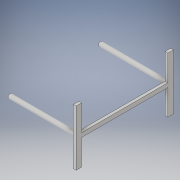
# Autodesk Inventor part: Spielstraßenschild_Teil_Unten
Saved by Autodesk Inventor 2019.5 (Build 235369000, 369)
## iProperties
Created: 2021-10-06
Part Number: Spielstraßenschild_Teil_Unten
Material: Generisch
Document SubType Name: Modeling
Designer: mritt
Density: 1 g/cm^3
Appearance: Vorgabe
Author: mritt
Autodesk Inventor part; units mm, degrees
ref_plane "YZ Plane" through (0, 0, 0) normal (1, 0, 0) x (0, 1, 0)
ref_plane "XZ Plane" through (0, 0, 0) normal (0, 1, 0) x (-1, 0, 0)
ref_plane "XY Plane" through (0, 0, 0) normal (0, 0, 1) x (1, 0, 0)
sketch "Skizze1" plane through (0, 0, 0) normal (0, 1, 0) x (-1, 0, 0)
  line L0 (37.9316, -16.2735) -> (-2.0684, -16.2735)
  line L1 (-2.0684, -16.2735) -> (-2.0684, -86.2735)
  line L2 (-2.0684, -86.2735) -> (37.9316, -86.2735)
  line L3 (37.9316, -86.2735) -> (37.9316, -16.2735)
  point P0 (0, 0)
  dimension "d0" = 70
  dimension "d1" = 40
  constraints: 8 end point, 2 parallel, 1 horizontal, 1 perpendicular
  measures "d0" distance of L2.end L0.start
  measures "d1" distance of L1.end L2.end
extrude "Extrusion1" add sketch "Skizze1" along normal blind 3
fillet "Rundung1" radius 1 4 edges at (-37.9316, 1.5, -16.2735) (-37.9316, 1.5, -86.2735) (2.0684, 1.5, -86.2735) (2.0684, 1.5, -16.2735)
sketch "Skizze2" plane through (2.0684, 0, -17.2735) normal (1, 0, 0) x (0, 0, -1)
  circle A0 centre (1.5, 1.5) radius 1.5
  circle A1 centre (66.5, 1.5) radius 1.5
  line L0 (0, 3) -> (68, 3) projected
  line L1 (0, 0) -> (0, 3) projected
  line L2 (68, 3) -> (68, 0) projected
  point P0 (-17.2735, 0)
  dimension "d5" = 3
  dimension "d6" = 3
  dimension "d7" = 1.5
  dimension "d8" = 1.5
  dimension "d9" = 1.5
  dimension "d10" = 1.5
  constraints: 2 centre point
  measures "d5" diameter of A0
  measures "d6" diameter of A1
  measures "d7" distance from line of A0.centre L0
  measures "d8" distance from line of A0.centre L1
  measures "d9" distance from line of A1.centre L0
  measures "d10" distance from line of L2 A1.centre
extrude "Extrusion2" add sketch "Skizze2" along normal blind 50 contours A0 | A1
sketch "Skizze3" plane through (52.0684, 1.5, -18.7735) normal (1, 0, 0) x (0, 0, -1)
  line L0 (-2.5, 1.5) -> (67.5, 1.5)
  line L1 (67.5, 1.5) -> (67.5, -1.5)
  line L2 (67.5, -1.5) -> (-2.5, -1.5)
  line L3 (-2.5, -1.5) -> (-2.5, 1.5)
  circle A0 centre (0, 0) radius 1.5 projected
  circle A1 centre (65, 0) radius 1.5 projected
  line L4 (-2.5, 20) -> (1.5, 20)
  line L5 (1.5, 20) -> (1.5, -20)
  line L6 (1.5, -20) -> (-2.5, -20)
  line L7 (-2.5, -20) -> (-2.5, 20)
  line L8 (67.5, 20) -> (63.5, 20)
  line L9 (63.5, 20) -> (63.5, -20)
  line L10 (63.5, -20) -> (67.5, -20)
  line L11 (67.5, -20) -> (67.5, 20)
  point P0 (-18.7735, -1.5)
  dimension "d13" = 1.5
  dimension "d14" = 1.5
  dimension "d16" = 2.5
  dimension "d17" = 2.5
  dimension "d20" = 40
  dimension "d21" = 20
  constraints: 24 end point, 6 parallel, 3 horizontal, 3 perpendicular, 2 collinear, 1 point on line
  measures "d13" distance from line of A0.centre L0
  measures "d14" distance from line of A0.centre L2
  measures "d16" distance from line of A0.centre L3
  measures "d17" distance from line of A1.centre L1
  measures "d20" distance of L6.end L4.start
  measures "d21" distance from line of A0.centre L4
extrude "Extrusion4" add sketch "Skizze3" against normal blind 2
sketch "Skizze4" plane through (0, 3, 0) normal (0, 1, 0) x (1, 0, 0)
  line L0 (2.0684, 14.6832) -> (-41.6445, 14.6832)
  line L1 (-41.6445, 14.6832) -> (-41.6445, 91.2635)
  line L2 (-41.6445, 91.2635) -> (2.0684, 91.2635)
  line L3 (2.0684, 91.2635) -> (2.0684, 14.6832)
  point P0 (0, 0)
  constraints: 8 end point, 2 parallel, 1 horizontal, 1 perpendicular
extrude "Extrusion5" cut sketch "Skizze4" against normal blind 10
